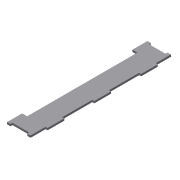
# Autodesk Inventor part: Frontal
Saved by Autodesk Inventor 2017 (Build 210142000, 142)
## iProperties
Created: 2017-06-23
Part Number: Frontal
Material: Generic
Document SubType Name: Modeling
Designer: Butri
Density: 1 g/cm^3
Appearance: Default
Author: Butri
Autodesk Inventor part; units mm, degrees
ref_plane "YZ Plane" through (0, 0, 0) normal (1, 0, 0) x (0, 1, 0)
ref_plane "XZ Plane" through (0, 0, 0) normal (0, 1, 0) x (-1, 0, 0)
ref_plane "XY Plane" through (0, 0, 0) normal (0, 0, 1) x (1, 0, 0)
sketch "Sketch1" plane through (0, 0, 0) normal (0, 0, 1) x (1, 0, 0)
  line L0 (-6, 375) -> (0, 375) construction
  line L1 (0, 375) -> (0, 420) construction
  line L2 (0, 420) -> (-6, 420) construction
  line L3 (-6, 375) -> (-6, 420) construction
  line L4 (-6, 235) -> (0, 235) construction
  line L5 (0, 235) -> (0, 325) construction
  line L6 (0, 325) -> (-6, 325) construction
  line L7 (-6, 235) -> (-6, 325) construction
  line L8 (0, 185) -> (-6, 185) construction
  line L9 (-6, 95) -> (-6, 185) construction
  line L10 (-6, 95) -> (0, 95) construction
  line L11 (0, 95) -> (0, 185) construction
  line L12 (0, 45) -> (-6, 45) construction
  line L13 (-6, 0) -> (-6, 45) construction
  line L14 (0, 0) -> (-6, 0) construction
  line L15 (0, 0) -> (0, 45) construction
  line L16 (-6, 375) -> (0, 375)
  line L17 (0, 375) -> (0, 325)
  line L18 (0, 325) -> (-6, 325)
  line L19 (-6, 235) -> (0, 235)
  line L20 (0, 235) -> (0, 185)
  line L21 (0, 185) -> (-6, 185)
  line L22 (-6, 95) -> (0, 95)
  line L23 (0, 95) -> (0, 45)
  line L24 (0, 45) -> (-6, 45)
  line L25 (-6, 0) -> (-6, 45)
  line L26 (-6, 95) -> (-6, 185)
  line L27 (-6, 235) -> (-6, 325)
  line L28 (-6, 375) -> (-6, 420)
  line L29 (-76, 375) -> (-61, 375)
  line L30 (-61, 375) -> (-61, 45)
  line L31 (-61, 45) -> (-76, 45)
  line L32 (-76, 420) -> (-76, 375)
  line L33 (-76, 45) -> (-76, 0)
  line L34 (-66, 420) -> (-66, 414)
  line L35 (-66, 414) -> (-16, 414)
  line L36 (-16, 414) -> (-16, 420)
  line L37 (0, 210) -> (-61, 210) construction
  line L38 (-66, 0) -> (-66, 6)
  line L39 (-66, 6) -> (-16, 6)
  line L40 (-16, 6) -> (-16, 0)
  line L41 (-76, 0) -> (-66, 0)
  line L42 (-16, 0) -> (-6, 0)
  line L43 (-6, 420) -> (-16, 420)
  line L44 (-66, 420) -> (-76, 420)
  dimension "d0" = 70
  dimension "d1" = 15
  dimension "d2" = 50
  dimension "d3" = 6
  dimension "d4" = 10
  constraints: 58 end point, 16 parallel, 9 perpendicular, 5 horizontal, 4 symmetric about line, 2 midpoint, 1 collinear
  measures "d0" distance of L25.start L33.end
  measures "d1" distance of L30.end L31.end
  measures "d2" distance of L35.end L34.end
  measures "d3" distance of L34.end L34.start
  measures "d4" distance between parallel lines of L32 L34
extrude "Extrusion1" add sketch "Sketch1" against normal blind 6
body "Solid1"
